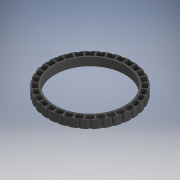
# Autodesk Inventor part: tsop_lid
Saved by Autodesk Inventor 2020 (Build 240168000, 168)
## iProperties
Created: 2024-11-04
Part Number: tsop_lid
Material: Полиэтилен, низкая плотность
Document SubType Name: Modeling
Designer: Ivan
Density: 0.894 g/cm^3
Appearance: Типовые
Mass: 11.4927 g
Surface Area: 157.828 cm^2
Volume: 12.8554 cm^3
Author: Ivan
Autodesk Inventor part; units mm, degrees
ref_plane "YZ Plane" through (0, 0, 0) normal (1, 0, 0) x (0, 1, 0)
ref_plane "XZ Plane" through (0, 0, 0) normal (0, 1, 0) x (-1, 0, 0)
ref_plane "XY Plane" through (0, 0, 0) normal (0, 0, 1) x (1, 0, 0)
sketch "Эскиз1" plane through (0, 0, 0) normal (0, 1, 0) x (-1, 0, 0)
  line L0 (48.127849, 3.6) -> (42.927849, 3.6)
  line L1 (42.927849, 3.6) -> (42.927849, -3.6)
  line L2 (42.927849, -3.6) -> (48.127849, -3.6)
  line L3 (48.127849, -3.6) -> (48.127849, 3.6)
  line L4 (0, 0) -> (42.927849, 0) construction
  circle A0 centre (0, 0) radius 45.669958 construction
  line L5 (45.527849, 3.6) -> (45.527849, -3.6) construction
  line L6 (41.400677, 11.905635) -> (42.805328, 4.843981)
  line L7 (46.500761, 12.920105) -> (41.400677, 11.905635)
  line L8 (47.905411, 5.858451) -> (46.500761, 12.920105)
  line L9 (42.805328, 4.843981) -> (47.905411, 5.858451)
  line L10 (38.282501, 19.753743) -> (41.037822, 13.10181)
  line L11 (43.086674, 21.743697) -> (38.282501, 19.753743)
  line L12 (45.841995, 15.091764) -> (43.086674, 21.743697)
  line L13 (41.037822, 13.10181) -> (45.841995, 15.091764)
  line L14 (33.693149, 26.842726) -> (37.693255, 20.856145)
  line L15 (38.016791, 29.731691) -> (33.693149, 26.842726)
  line L16 (42.016897, 23.74511) -> (38.016791, 29.731691)
  line L17 (37.693255, 20.856145) -> (42.016897, 23.74511)
  line L18 (27.808989, 32.900158) -> (32.900158, 27.808989)
  line L19 (31.485944, 36.577113) -> (27.808989, 32.900158)
  line L20 (36.577113, 31.485944) -> (31.485944, 36.577113)
  line L21 (32.900158, 27.808989) -> (36.577113, 31.485944)
  line L22 (20.856145, 37.693255) -> (26.842726, 33.693149)
  line L23 (23.74511, 42.016897) -> (20.856145, 37.693255)
  line L24 (29.731691, 38.016791) -> (23.74511, 42.016897)
  line L25 (26.842726, 33.693149) -> (29.731691, 38.016791)
  line L26 (13.10181, 41.037822) -> (19.753743, 38.282501)
  line L27 (15.091764, 45.841995) -> (13.10181, 41.037822)
  line L28 (21.743697, 43.086674) -> (15.091764, 45.841995)
  line L29 (19.753743, 38.282501) -> (21.743697, 43.086674)
  line L30 (4.843981, 42.805328) -> (11.905635, 41.400677)
  line L31 (5.858451, 47.905411) -> (4.843981, 42.805328)
  line L32 (12.920105, 46.500761) -> (5.858451, 47.905411)
  line L33 (11.905635, 41.400677) -> (12.920105, 46.500761)
  line L34 (-3.6, 42.927849) -> (3.6, 42.927849)
  line L35 (-3.6, 48.127849) -> (-3.6, 42.927849)
  line L36 (3.6, 48.127849) -> (-3.6, 48.127849)
  line L37 (3.6, 42.927849) -> (3.6, 48.127849)
  line L38 (-11.905635, 41.400677) -> (-4.843981, 42.805328)
  line L39 (-12.920105, 46.500761) -> (-11.905635, 41.400677)
  line L40 (-5.858451, 47.905411) -> (-12.920105, 46.500761)
  line L41 (-4.843981, 42.805328) -> (-5.858451, 47.905411)
  line L42 (-19.753743, 38.282501) -> (-13.10181, 41.037822)
  line L43 (-21.743697, 43.086674) -> (-19.753743, 38.282501)
  line L44 (-15.091764, 45.841995) -> (-21.743697, 43.086674)
  line L45 (-13.10181, 41.037822) -> (-15.091764, 45.841995)
  line L46 (-26.842726, 33.693149) -> (-20.856145, 37.693255)
  line L47 (-29.731691, 38.016791) -> (-26.842726, 33.693149)
  line L48 (-23.74511, 42.016897) -> (-29.731691, 38.016791)
  line L49 (-20.856145, 37.693255) -> (-23.74511, 42.016897)
  line L50 (-32.900158, 27.808989) -> (-27.808989, 32.900158)
  line L51 (-36.577113, 31.485944) -> (-32.900158, 27.808989)
  line L52 (-31.485944, 36.577113) -> (-36.577113, 31.485944)
  line L53 (-27.808989, 32.900158) -> (-31.485944, 36.577113)
  line L54 (-37.693255, 20.856145) -> (-33.693149, 26.842726)
  line L55 (-42.016897, 23.74511) -> (-37.693255, 20.856145)
  line L56 (-38.016791, 29.731691) -> (-42.016897, 23.74511)
  line L57 (-33.693149, 26.842726) -> (-38.016791, 29.731691)
  line L58 (-41.037822, 13.10181) -> (-38.282501, 19.753743)
  line L59 (-45.841995, 15.091764) -> (-41.037822, 13.10181)
  line L60 (-43.086674, 21.743697) -> (-45.841995, 15.091764)
  line L61 (-38.282501, 19.753743) -> (-43.086674, 21.743697)
  line L62 (-42.805328, 4.843981) -> (-41.400677, 11.905635)
  line L63 (-47.905411, 5.858451) -> (-42.805328, 4.843981)
  line L64 (-46.500761, 12.920105) -> (-47.905411, 5.858451)
  line L65 (-41.400677, 11.905635) -> (-46.500761, 12.920105)
  line L66 (-42.927849, -3.6) -> (-42.927849, 3.6)
  line L67 (-48.127849, -3.6) -> (-42.927849, -3.6)
  line L68 (-48.127849, 3.6) -> (-48.127849, -3.6)
  line L69 (-42.927849, 3.6) -> (-48.127849, 3.6)
  line L70 (-41.400677, -11.905635) -> (-42.805328, -4.843981)
  line L71 (-46.500761, -12.920105) -> (-41.400677, -11.905635)
  line L72 (-47.905411, -5.858451) -> (-46.500761, -12.920105)
  line L73 (-42.805328, -4.843981) -> (-47.905411, -5.858451)
  line L74 (-38.282501, -19.753743) -> (-41.037822, -13.10181)
  line L75 (-43.086674, -21.743697) -> (-38.282501, -19.753743)
  line L76 (-45.841995, -15.091764) -> (-43.086674, -21.743697)
  line L77 (-41.037822, -13.10181) -> (-45.841995, -15.091764)
  line L78 (-33.693149, -26.842726) -> (-37.693255, -20.856145)
  line L79 (-38.016791, -29.731691) -> (-33.693149, -26.842726)
  line L80 (-42.016897, -23.74511) -> (-38.016791, -29.731691)
  line L81 (-37.693255, -20.856145) -> (-42.016897, -23.74511)
  line L82 (-27.808989, -32.900158) -> (-32.900158, -27.808989)
  line L83 (-31.485944, -36.577113) -> (-27.808989, -32.900158)
  line L84 (-36.577113, -31.485944) -> (-31.485944, -36.577113)
  line L85 (-32.900158, -27.808989) -> (-36.577113, -31.485944)
  line L86 (-20.856145, -37.693255) -> (-26.842726, -33.693149)
  line L87 (-23.74511, -42.016897) -> (-20.856145, -37.693255)
  line L88 (-29.731691, -38.016791) -> (-23.74511, -42.016897)
  line L89 (-26.842726, -33.693149) -> (-29.731691, -38.016791)
  line L90 (-13.10181, -41.037822) -> (-19.753743, -38.282501)
  line L91 (-15.091764, -45.841995) -> (-13.10181, -41.037822)
  line L92 (-21.743697, -43.086674) -> (-15.091764, -45.841995)
  line L93 (-19.753743, -38.282501) -> (-21.743697, -43.086674)
  line L94 (-4.843981, -42.805328) -> (-11.905635, -41.400677)
  line L95 (-5.858451, -47.905411) -> (-4.843981, -42.805328)
  line L96 (-12.920105, -46.500761) -> (-5.858451, -47.905411)
  line L97 (-11.905635, -41.400677) -> (-12.920105, -46.500761)
  line L98 (3.6, -42.927849) -> (-3.6, -42.927849)
  line L99 (3.6, -48.127849) -> (3.6, -42.927849)
  line L100 (-3.6, -48.127849) -> (3.6, -48.127849)
  line L101 (-3.6, -42.927849) -> (-3.6, -48.127849)
  line L102 (11.905635, -41.400677) -> (4.843981, -42.805328)
  line L103 (12.920105, -46.500761) -> (11.905635, -41.400677)
  line L104 (5.858451, -47.905411) -> (12.920105, -46.500761)
  line L105 (4.843981, -42.805328) -> (5.858451, -47.905411)
  line L106 (19.753743, -38.282501) -> (13.10181, -41.037822)
  line L107 (21.743697, -43.086674) -> (19.753743, -38.282501)
  line L108 (15.091764, -45.841995) -> (21.743697, -43.086674)
  line L109 (13.10181, -41.037822) -> (15.091764, -45.841995)
  line L110 (26.842726, -33.693149) -> (20.856145, -37.693255)
  line L111 (29.731691, -38.016791) -> (26.842726, -33.693149)
  line L112 (23.74511, -42.016897) -> (29.731691, -38.016791)
  line L113 (20.856145, -37.693255) -> (23.74511, -42.016897)
  line L114 (32.900158, -27.808989) -> (27.808989, -32.900158)
  line L115 (36.577113, -31.485944) -> (32.900158, -27.808989)
  line L116 (31.485944, -36.577113) -> (36.577113, -31.485944)
  line L117 (27.808989, -32.900158) -> (31.485944, -36.577113)
  line L118 (37.693255, -20.856145) -> (33.693149, -26.842726)
  line L119 (42.016897, -23.74511) -> (37.693255, -20.856145)
  line L120 (38.016791, -29.731691) -> (42.016897, -23.74511)
  line L121 (33.693149, -26.842726) -> (38.016791, -29.731691)
  line L122 (41.037822, -13.10181) -> (38.282501, -19.753743)
  line L123 (45.841995, -15.091764) -> (41.037822, -13.10181)
  line L124 (43.086674, -21.743697) -> (45.841995, -15.091764)
  line L125 (38.282501, -19.753743) -> (43.086674, -21.743697)
  line L126 (42.805328, -4.843981) -> (41.400677, -11.905635)
  line L127 (47.905411, -5.858451) -> (42.805328, -4.843981)
  line L128 (46.500761, -12.920105) -> (47.905411, -5.858451)
  line L129 (41.400677, -11.905635) -> (46.500761, -12.920105)
  line L130 (42.805328, 4.843981) -> (42.927849, 3.6) construction
  line L131 (42.927849, 3.6) -> (46.884011, 3.989648) construction
  point P0 (45.669958, 0)
  point P1 (42.103003, 8.374808)
  point P2 (43.950719, 12.41287)
  point P3 (45.355369, 5.351216)
  point P4 (39.660161, 16.427777)
  point P5 (40.684588, 20.74872)
  point P6 (43.439908, 14.096787)
  point P7 (35.693202, 23.849435)
  point P8 (35.85497, 28.287208)
  point P9 (39.855076, 22.300627)
  point P10 (30.354573, 30.354573)
  point P11 (29.647466, 34.738635)
  point P12 (34.738635, 29.647466)
  point P13 (23.849435, 35.693202)
  point P14 (22.300627, 39.855076)
  point P15 (28.287208, 35.85497)
  point P16 (16.427777, 39.660161)
  point P17 (14.096787, 43.439908)
  point P18 (20.74872, 40.684588)
  point P19 (8.374808, 42.103003)
  point P20 (5.351216, 45.355369)
  point P21 (12.41287, 43.950719)
  point P22 (0, 42.927849)
  point P23 (-3.6, 45.527849)
  point P24 (3.6, 45.527849)
  point P25 (-8.374808, 42.103003)
  point P26 (-12.41287, 43.950719)
  point P27 (-5.351216, 45.355369)
  point P28 (-16.427777, 39.660161)
  point P29 (-20.74872, 40.684588)
  point P30 (-14.096787, 43.439908)
  point P31 (-23.849435, 35.693202)
  point P32 (-28.287208, 35.85497)
  point P33 (-22.300627, 39.855076)
  point P34 (-30.354573, 30.354573)
  point P35 (-34.738635, 29.647466)
  point P36 (-29.647466, 34.738635)
  point P37 (-35.693202, 23.849435)
  point P38 (-39.855076, 22.300627)
  point P39 (-35.85497, 28.287208)
  point P40 (-39.660161, 16.427777)
  point P41 (-43.439908, 14.096787)
  point P42 (-40.684588, 20.74872)
  point P43 (-42.103003, 8.374808)
  point P44 (-45.355369, 5.351216)
  point P45 (-43.950719, 12.41287)
  point P46 (-42.927849, 0)
  point P47 (-45.527849, -3.6)
  point P48 (-45.527849, 3.6)
  point P49 (-42.103003, -8.374808)
  point P50 (-43.950719, -12.41287)
  point P51 (-45.355369, -5.351216)
  point P52 (-39.660161, -16.427777)
  point P53 (-40.684588, -20.74872)
  point P54 (-43.439908, -14.096787)
  point P55 (-35.693202, -23.849435)
  point P56 (-35.85497, -28.287208)
  point P57 (-39.855076, -22.300627)
  point P58 (-30.354573, -30.354573)
  point P59 (-29.647466, -34.738635)
  point P60 (-34.738635, -29.647466)
  point P61 (-23.849435, -35.693202)
  point P62 (-22.300627, -39.855076)
  point P63 (-28.287208, -35.85497)
  point P64 (-16.427777, -39.660161)
  point P65 (-14.096787, -43.439908)
  point P66 (-20.74872, -40.684588)
  point P67 (-8.374808, -42.103003)
  point P68 (-5.351216, -45.355369)
  point P69 (-12.41287, -43.950719)
  point P70 (0, -42.927849)
  point P71 (3.6, -45.527849)
  point P72 (-3.6, -45.527849)
  point P73 (8.374808, -42.103003)
  point P74 (12.41287, -43.950719)
  point P75 (5.351216, -45.355369)
  point P76 (16.427777, -39.660161)
  point P77 (20.74872, -40.684588)
  point P78 (14.096787, -43.439908)
  point P79 (23.849435, -35.693202)
  point P80 (28.287208, -35.85497)
  point P81 (22.300627, -39.855076)
  point P82 (30.354573, -30.354573)
  point P83 (34.738635, -29.647466)
  point P84 (29.647466, -34.738635)
  point P85 (35.693202, -23.849435)
  point P86 (39.855076, -22.300627)
  point P87 (35.85497, -28.287208)
  point P88 (39.660161, -16.427777)
  point P89 (43.439908, -14.096787)
  point P90 (40.684588, -20.74872)
  point P91 (42.103003, -8.374808)
  point P92 (45.355369, -5.351216)
  point P93 (43.950719, -12.41287)
  dimension "d0" = 7.2
  dimension "d1" = 5.2
  dimension "d5" = 360
  dimension "d7" = 1.25
  constraints: 262 end point, 33 midpoint, 3 point on circle, 2 horizontal, 2 perpendicular, 1 centre point, 1 coincident, 1 parallel, 1 point on line, 1 vertical, 357 other
  measures "d0" distance of L1.start L1.end
  measures "d1" distance from line of L1 L2.end
  measures "d7" distance from line of L131 L6.end
sketch "Эскиз3" plane through (0, 0, 0) normal (0, 1, 0) x (-1, 0, 0)
  line L0 (42.805328, 4.843981) -> (42.927849, 3.6) construction
  line L1 (42.866588, 4.22199) -> (50.472791, 4.971136) construction
  line L2 (48.127849, -3.6) -> (48.127849, 3.6)
  line L3 (48.127849, -0.05) -> (48.127849, 0.05)
  line L4 (48.127849, 2.45) -> (49.327849, 2.45) construction
  arc A0 (48.127849, 0.05) -> (49.327849, 2.45) centre (46.327849, 2.45) ccw
  line L5 (49.327849, 2.45) -> (49.327849, 0) construction
  line L6 (0, 0) -> (42.927849, 0) construction
  arc A1 (49.327849, -2.45) -> (48.127849, -0.05) centre (46.327849, -2.45) ccw
  arc A2 (47.193332, 9.438317) -> (47.902057, 12.02631) centre (44.959701, 11.441039) ccw
  arc A3 (48.858, 7.220462) -> (47.212841, 9.340238) centre (45.915644, 6.635191) ccw
  line L7 (47.212841, 9.340238) -> (47.193332, 9.438317)
  arc A4 (44.445201, 18.463924) -> (44.635416, 21.140455) centre (41.863777, 19.992405) ccw
  arc A5 (46.510565, 16.613446) -> (44.483469, 18.371537) centre (43.738926, 15.465395) ccw
  line L8 (44.483469, 18.371537) -> (44.445201, 18.463924)
  arc A6 (39.989066, 26.779974) -> (39.653461, 29.442185) centre (37.159052, 27.775475) ccw
  arc A7 (42.375755, 25.367984) -> (40.044623, 26.696827) centre (39.881346, 23.701273) ccw
  line L9 (40.044623, 26.696827) -> (39.989066, 26.779974)
  arc A8 (33.996173, 34.066884) -> (33.147645, 36.612468) centre (31.026325, 34.491148) ccw
  arc A9 (36.612468, 33.147645) -> (34.066884, 33.996173) centre (34.491148, 31.026325) ccw
  line L10 (34.066884, 33.996173) -> (33.996173, 34.066884)
  arc A10 (26.696827, 40.044623) -> (25.367984, 42.375755) centre (23.701273, 39.881346) ccw
  arc A11 (29.442185, 39.653461) -> (26.779974, 39.989066) centre (27.775475, 37.159052) ccw
  line L11 (26.779974, 39.989066) -> (26.696827, 40.044623)
  arc A12 (18.371537, 44.483469) -> (16.613446, 46.510565) centre (15.465395, 43.738926) ccw
  arc A13 (21.140455, 44.635416) -> (18.463924, 44.445201) centre (19.992405, 41.863777) ccw
  line L12 (18.463924, 44.445201) -> (18.371537, 44.483469)
  arc A14 (9.340238, 47.212841) -> (7.220462, 48.858) centre (6.635191, 45.915644) ccw
  arc A15 (12.02631, 47.902057) -> (9.438317, 47.193332) centre (11.441039, 44.959701) ccw
  line L13 (9.438317, 47.193332) -> (9.340238, 47.212841)
  arc A16 (-0.05, 48.127849) -> (-2.45, 49.327849) centre (-2.45, 46.327849) ccw
  arc A17 (2.45, 49.327849) -> (0.05, 48.127849) centre (2.45, 46.327849) ccw
  line L14 (0.05, 48.127849) -> (-0.05, 48.127849)
  arc A18 (-9.438317, 47.193332) -> (-12.02631, 47.902057) centre (-11.441039, 44.959701) ccw
  arc A19 (-7.220462, 48.858) -> (-9.340238, 47.212841) centre (-6.635191, 45.915644) ccw
  line L15 (-9.340238, 47.212841) -> (-9.438317, 47.193332)
  arc A20 (-18.463924, 44.445201) -> (-21.140455, 44.635416) centre (-19.992405, 41.863777) ccw
  arc A21 (-16.613446, 46.510565) -> (-18.371537, 44.483469) centre (-15.465395, 43.738926) ccw
  line L16 (-18.371537, 44.483469) -> (-18.463924, 44.445201)
  arc A22 (-26.779974, 39.989066) -> (-29.442185, 39.653461) centre (-27.775475, 37.159052) ccw
  arc A23 (-25.367984, 42.375755) -> (-26.696827, 40.044623) centre (-23.701273, 39.881346) ccw
  line L17 (-26.696827, 40.044623) -> (-26.779974, 39.989066)
  arc A24 (-34.066884, 33.996173) -> (-36.612468, 33.147645) centre (-34.491148, 31.026325) ccw
  arc A25 (-33.147645, 36.612468) -> (-33.996173, 34.066884) centre (-31.026325, 34.491148) ccw
  line L18 (-33.996173, 34.066884) -> (-34.066884, 33.996173)
  arc A26 (-40.044623, 26.696827) -> (-42.375755, 25.367984) centre (-39.881346, 23.701273) ccw
  arc A27 (-39.653461, 29.442185) -> (-39.989066, 26.779974) centre (-37.159052, 27.775475) ccw
  line L19 (-39.989066, 26.779974) -> (-40.044623, 26.696827)
  arc A28 (-44.483469, 18.371537) -> (-46.510565, 16.613446) centre (-43.738926, 15.465395) ccw
  arc A29 (-44.635416, 21.140455) -> (-44.445201, 18.463924) centre (-41.863777, 19.992405) ccw
  line L20 (-44.445201, 18.463924) -> (-44.483469, 18.371537)
  arc A30 (-47.212841, 9.340238) -> (-48.858, 7.220462) centre (-45.915644, 6.635191) ccw
  arc A31 (-47.902057, 12.02631) -> (-47.193332, 9.438317) centre (-44.959701, 11.441039) ccw
  line L21 (-47.193332, 9.438317) -> (-47.212841, 9.340238)
  arc A32 (-48.127849, -0.05) -> (-49.327849, -2.45) centre (-46.327849, -2.45) ccw
  arc A33 (-49.327849, 2.45) -> (-48.127849, 0.05) centre (-46.327849, 2.45) ccw
  line L22 (-48.127849, 0.05) -> (-48.127849, -0.05)
  arc A34 (-47.193332, -9.438317) -> (-47.902057, -12.02631) centre (-44.959701, -11.441039) ccw
  arc A35 (-48.858, -7.220462) -> (-47.212841, -9.340238) centre (-45.915644, -6.635191) ccw
  line L23 (-47.212841, -9.340238) -> (-47.193332, -9.438317)
  arc A36 (-44.445201, -18.463924) -> (-44.635416, -21.140455) centre (-41.863777, -19.992405) ccw
  arc A37 (-46.510565, -16.613446) -> (-44.483469, -18.371537) centre (-43.738926, -15.465395) ccw
  line L24 (-44.483469, -18.371537) -> (-44.445201, -18.463924)
  arc A38 (-39.989066, -26.779974) -> (-39.653461, -29.442185) centre (-37.159052, -27.775475) ccw
  arc A39 (-42.375755, -25.367984) -> (-40.044623, -26.696827) centre (-39.881346, -23.701273) ccw
  line L25 (-40.044623, -26.696827) -> (-39.989066, -26.779974)
  arc A40 (-33.996173, -34.066884) -> (-33.147645, -36.612468) centre (-31.026325, -34.491148) ccw
  arc A41 (-36.612468, -33.147645) -> (-34.066884, -33.996173) centre (-34.491148, -31.026325) ccw
  line L26 (-34.066884, -33.996173) -> (-33.996173, -34.066884)
  arc A42 (-26.696827, -40.044623) -> (-25.367984, -42.375755) centre (-23.701273, -39.881346) ccw
  arc A43 (-29.442185, -39.653461) -> (-26.779974, -39.989066) centre (-27.775475, -37.159052) ccw
  line L27 (-26.779974, -39.989066) -> (-26.696827, -40.044623)
  arc A44 (-18.371537, -44.483469) -> (-16.613446, -46.510565) centre (-15.465395, -43.738926) ccw
  arc A45 (-21.140455, -44.635416) -> (-18.463924, -44.445201) centre (-19.992405, -41.863777) ccw
  line L28 (-18.463924, -44.445201) -> (-18.371537, -44.483469)
  arc A46 (-9.340238, -47.212841) -> (-7.220462, -48.858) centre (-6.635191, -45.915644) ccw
  arc A47 (-12.02631, -47.902057) -> (-9.438317, -47.193332) centre (-11.441039, -44.959701) ccw
  line L29 (-9.438317, -47.193332) -> (-9.340238, -47.212841)
  arc A48 (0.05, -48.127849) -> (2.45, -49.327849) centre (2.45, -46.327849) ccw
  arc A49 (-2.45, -49.327849) -> (-0.05, -48.127849) centre (-2.45, -46.327849) ccw
  line L30 (-0.05, -48.127849) -> (0.05, -48.127849)
  arc A50 (9.438317, -47.193332) -> (12.02631, -47.902057) centre (11.441039, -44.959701) ccw
  arc A51 (7.220462, -48.858) -> (9.340238, -47.212841) centre (6.635191, -45.915644) ccw
  line L31 (9.340238, -47.212841) -> (9.438317, -47.193332)
  arc A52 (18.463924, -44.445201) -> (21.140455, -44.635416) centre (19.992405, -41.863777) ccw
  arc A53 (16.613446, -46.510565) -> (18.371537, -44.483469) centre (15.465395, -43.738926) ccw
  line L32 (18.371537, -44.483469) -> (18.463924, -44.445201)
  arc A54 (26.779974, -39.989066) -> (29.442185, -39.653461) centre (27.775475, -37.159052) ccw
  arc A55 (25.367984, -42.375755) -> (26.696827, -40.044623) centre (23.701273, -39.881346) ccw
  line L33 (26.696827, -40.044623) -> (26.779974, -39.989066)
  arc A56 (34.066884, -33.996173) -> (36.612468, -33.147645) centre (34.491148, -31.026325) ccw
  arc A57 (33.147645, -36.612468) -> (33.996173, -34.066884) centre (31.026325, -34.491148) ccw
  line L34 (33.996173, -34.066884) -> (34.066884, -33.996173)
  arc A58 (40.044623, -26.696827) -> (42.375755, -25.367984) centre (39.881346, -23.701273) ccw
  arc A59 (39.653461, -29.442185) -> (39.989066, -26.779974) centre (37.159052, -27.775475) ccw
  line L35 (39.989066, -26.779974) -> (40.044623, -26.696827)
  arc A60 (44.483469, -18.371537) -> (46.510565, -16.613446) centre (43.738926, -15.465395) ccw
  arc A61 (44.635416, -21.140455) -> (44.445201, -18.463924) centre (41.863777, -19.992405) ccw
  line L36 (44.445201, -18.463924) -> (44.483469, -18.371537)
  arc A62 (47.212841, -9.340238) -> (48.858, -7.220462) centre (45.915644, -6.635191) ccw
  arc A63 (47.902057, -12.02631) -> (47.193332, -9.438317) centre (44.959701, -11.441039) ccw
  line L37 (47.193332, -9.438317) -> (47.212841, -9.340238)
  arc A64 (49.327849, 2.45) -> (48.858, 7.220462) centre (0, 0) ccw
  arc A65 (47.902057, 12.02631) -> (46.510565, 16.613446) centre (0, 0) ccw
  arc A66 (44.635416, 21.140455) -> (42.375755, 25.367984) centre (0, 0) ccw
  arc A67 (39.653461, 29.442185) -> (36.612468, 33.147645) centre (0, 0) ccw
  arc A68 (33.147645, 36.612468) -> (29.442185, 39.653461) centre (0, 0) ccw
  arc A69 (25.367984, 42.375755) -> (21.140455, 44.635416) centre (0, 0) ccw
  arc A70 (16.613446, 46.510565) -> (12.02631, 47.902057) centre (0, 0) ccw
  arc A71 (7.220462, 48.858) -> (2.45, 49.327849) centre (0, 0) ccw
  arc A72 (-2.45, 49.327849) -> (-7.220462, 48.858) centre (0, 0) ccw
  arc A73 (-12.02631, 47.902057) -> (-16.613446, 46.510565) centre (0, 0) ccw
  arc A74 (-21.140455, 44.635416) -> (-25.367984, 42.375755) centre (0, 0) ccw
  arc A75 (-29.442185, 39.653461) -> (-33.147645, 36.612468) centre (0, 0) ccw
  arc A76 (-36.612468, 33.147645) -> (-39.653461, 29.442185) centre (0, 0) ccw
  arc A77 (-42.375755, 25.367984) -> (-44.635416, 21.140455) centre (0, 0) ccw
  arc A78 (-46.510565, 16.613446) -> (-47.902057, 12.02631) centre (0, 0) ccw
  arc A79 (-48.858, 7.220462) -> (-49.327849, 2.45) centre (0, 0) ccw
  arc A80 (-49.327849, -2.45) -> (-48.858, -7.220462) centre (0, 0) ccw
  arc A81 (-47.902057, -12.02631) -> (-46.510565, -16.613446) centre (0, 0) ccw
  arc A82 (-44.635416, -21.140455) -> (-42.375755, -25.367984) centre (0, 0) ccw
  arc A83 (-39.653461, -29.442185) -> (-36.612468, -33.147645) centre (0, 0) ccw
  arc A84 (-33.147645, -36.612468) -> (-29.442185, -39.653461) centre (0, 0) ccw
  arc A85 (-25.367984, -42.375755) -> (-21.140455, -44.635416) centre (0, 0) ccw
  arc A86 (-16.613446, -46.510565) -> (-12.02631, -47.902057) centre (0, 0) ccw
  arc A87 (-7.220462, -48.858) -> (-2.45, -49.327849) centre (0, 0) ccw
  arc A88 (2.45, -49.327849) -> (7.220462, -48.858) centre (0, 0) ccw
  arc A89 (12.02631, -47.902057) -> (16.613446, -46.510565) centre (0, 0) ccw
  arc A90 (21.140455, -44.635416) -> (25.367984, -42.375755) centre (0, 0) ccw
  arc A91 (29.442185, -39.653461) -> (33.147645, -36.612468) centre (0, 0) ccw
  arc A92 (36.612468, -33.147645) -> (39.653461, -29.442185) centre (0, 0) ccw
  arc A93 (42.375755, -25.367984) -> (44.635416, -21.140455) centre (0, 0) ccw
  arc A94 (46.510565, -16.613446) -> (47.902057, -12.02631) centre (0, 0) ccw
  arc A95 (48.858, -7.220462) -> (49.327849, -2.45) centre (0, 0) ccw
  circle A96 centre (0, 0) radius 40.927849
  line L38 (42.927849, 3.6) -> (42.927849, -3.6)
  point P0 (48.127849, 0)
  point P1 (47.203086, 9.389278)
  point P2 (44.464335, 18.417731)
  point P3 (40.016844, 26.7384)
  point P4 (34.031529, 34.031529)
  point P5 (26.7384, 40.016844)
  point P6 (18.417731, 44.464335)
  point P7 (9.389278, 47.203086)
  point P8 (0, 48.127849)
  point P9 (-9.389278, 47.203086)
  point P10 (-18.417731, 44.464335)
  point P11 (-26.7384, 40.016844)
  point P12 (-34.031529, 34.031529)
  point P13 (-40.016844, 26.7384)
  point P14 (-44.464335, 18.417731)
  point P15 (-47.203086, 9.389278)
  point P16 (-48.127849, 0)
  point P17 (-47.203086, -9.389278)
  point P18 (-44.464335, -18.417731)
  point P19 (-40.016844, -26.7384)
  point P20 (-34.031529, -34.031529)
  point P21 (-26.7384, -40.016844)
  point P22 (-18.417731, -44.464335)
  point P23 (-9.389278, -47.203086)
  point P24 (0, -48.127849)
  point P25 (9.389278, -47.203086)
  point P26 (18.417731, -44.464335)
  point P27 (26.7384, -40.016844)
  point P28 (34.031529, -34.031529)
  point P29 (40.016844, -26.7384)
  point P30 (44.464335, -18.417731)
  point P31 (47.203086, -9.389278)
  point P32 (40.927849, 0)
  point P33 (48.858, -7.220462)
  point P34 (49.327849, -2.45)
  point P35 (48.127849, -0.05)
  point P36 (48.127849, 0.05)
  point P37 (47.902057, 12.02631)
  point P38 (46.510565, 16.613446)
  point P39 (44.635416, 21.140455)
  point P40 (42.375755, 25.367984)
  point P41 (39.653461, 29.442185)
  point P42 (36.612468, 33.147645)
  point P43 (33.147645, 36.612468)
  point P44 (29.442185, 39.653461)
  point P45 (25.367984, 42.375755)
  point P46 (21.140455, 44.635416)
  point P47 (16.613446, 46.510565)
  point P48 (12.02631, 47.902057)
  point P49 (7.220462, 48.858)
  point P50 (2.45, 49.327849)
  point P51 (-2.45, 49.327849)
  point P52 (-7.220462, 48.858)
  point P53 (-12.02631, 47.902057)
  point P54 (-16.613446, 46.510565)
  point P55 (-21.140455, 44.635416)
  point P56 (-25.367984, 42.375755)
  point P57 (-29.442185, 39.653461)
  point P58 (-33.147645, 36.612468)
  point P59 (-36.612468, 33.147645)
  point P60 (-39.653461, 29.442185)
  point P61 (-42.375755, 25.367984)
  point P62 (-44.635416, 21.140455)
  point P63 (-46.510565, 16.613446)
  point P64 (-47.902057, 12.02631)
  point P65 (-48.858, 7.220462)
  point P66 (-49.327849, 2.45)
  point P67 (-49.327849, -2.45)
  point P68 (-48.858, -7.220462)
  point P69 (-47.902057, -12.02631)
  point P70 (-46.510565, -16.613446)
  point P71 (-44.635416, -21.140455)
  point P72 (-42.375755, -25.367984)
  point P73 (-39.653461, -29.442185)
  point P74 (-36.612468, -33.147645)
  point P75 (-33.147645, -36.612468)
  point P76 (-29.442185, -39.653461)
  point P77 (-25.367984, -42.375755)
  point P78 (-21.140455, -44.635416)
  point P79 (-16.613446, -46.510565)
  point P80 (-12.02631, -47.902057)
  point P81 (-7.220462, -48.858)
  point P82 (-2.45, -49.327849)
  point P83 (2.45, -49.327849)
  point P84 (7.220462, -48.858)
  point P85 (12.02631, -47.902057)
  point P86 (16.613446, -46.510565)
  point P87 (21.140455, -44.635416)
  point P88 (25.367984, -42.375755)
  point P89 (29.442185, -39.653461)
  point P90 (33.147645, -36.612468)
  point P91 (36.612468, -33.147645)
  point P92 (39.653461, -29.442185)
  point P93 (42.375755, -25.367984)
  point P94 (44.635416, -21.140455)
  point P95 (46.510565, -16.613446)
  point P96 (47.902057, -12.02631)
  dimension "d25" = 0.1
  dimension "d26" = 1.2
  dimension "d29" = 2.4
  dimension "d32" = 360
  dimension "d36" = 360
  dimension "d38" = 2
  constraints: 192 point on circle, 96 centre point, 70 end point, 4 point on line, 2 coincident, 2 midpoint, 2 perpendicular, 2 symmetric about line, 1 collinear, 1 horizontal, 1 horizontal alignment, 1 tangent, 453 other
  measures "d25" distance of L3.start L3.end
  measures "d26" distance of L4.start L4.end
  measures "d29" distance from line of L4 L3.end
  measures "d38" distance from line of L38 point (40.928, 0)
extrude "Выдавливание4" add sketch "Эскиз3" along normal blind 7.2
extrude "Выдавливание3" cut sketch "Эскиз1" along normal through all
extrude "Выдавливание5" add sketch "Эскиз3" against normal blind 2
equation "\"d29\" = 2 * d26"
